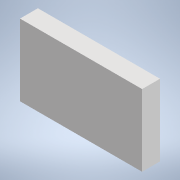
# Autodesk Inventor part: ESC
Saved by Autodesk Inventor 2020 (Build 240168000, 168)
## iProperties
Created: 2019-06-17
Part Number: ESC
Material: Generic
Document SubType Name: Modeling
Designer: amirt
Density: 1 g/cm^3
Appearance: Default
Author: amirt
Autodesk Inventor part; units mm, degrees
ref_plane "YZ Plane" through (0, 0, 0) normal (1, 0, 0) x (0, 1, 0)
ref_plane "XZ Plane" through (0, 0, 0) normal (0, 1, 0) x (-1, 0, 0)
ref_plane "XY Plane" through (0, 0, 0) normal (0, 0, 1) x (1, 0, 0)
sketch "Sketch1" plane through (0, 0, 0) normal (0, 0, 1) x (1, 0, 0)
  circle A0 centre (65.7667, 0.0011) radius 1.1 projected
  line L0 (-36.8269, 0.1559) -> (-36.8269, -12.5441)
  line L1 (-36.8269, -12.5441) -> (0, -12.5441)
  line L2 (0, 12.7) -> (-36.8269, 12.7)
  line L3 (-36.8269, 12.7) -> (-36.8269, -12.5441)
  line L4 (-36.8269, -12.5441) -> (13.9731, -12.5441)
  line L5 (13.9731, -12.5441) -> (13.9731, 12.7)
  line L6 (13.9731, 12.7) -> (-36.8269, 12.7)
  line L7 (-36.8269, 12.7) -> (-36.8269, -12.5441)
  point P0 (0, 0)
  dimension "d0" = 12.7
  dimension "d1" = 12.7
  dimension "d4" = 50.8
  constraints: 16 end point, 3 parallel, 2 horizontal, 1 perpendicular
  measures "d0" distance of L0.start L0.end
  measures "d1" distance of point (0, 0) L2.start
  measures "d4" distance of L6.end L5.end
extrude "Extrusion2" add sketch "Sketch1" along normal blind 6.35 contours L3 L2 L6 L5 L4 L1 L0
body "Solid2"
